7540a58a-294f-455a-a0d2-f9cc7533da06 (Autodesk Fusion 360 design; units mm, degrees)
Autodesk Fusion 360 part; units mm, degrees
note: some values were not read from the file. Set by a fixed rule: which sketch regions a step uses.
sketch "Sketch1" plane through (0, 0, 0) normal (0, 1, 0) x (1, 0, 0)
  circle A0 centre (0, 0) radius 16.9291
  circle A1 centre (0, 0) radius 19.05
  circle A2 centre (0, 0) radius 15.518342
  circle A3 centre (0, 0) radius 15.90815
  arc A4 (19.001185, -1.362896) -> (-17.460766, -7.617357) centre (0, 0) ccw
  circle A5 centre (0, 0) radius 1.984375
  line L0 (0, 0) -> (19.05, 0) construction
  line L1 (0, 0) -> (-1.386487, -15.847615)
  line L2 (0, 0) -> (-2.762421, -15.66647)
  line L3 (0, 0) -> (-4.117332, -15.366093)
  line L4 (0, 0) -> (-5.440908, -14.948771)
  line L5 (0, 0) -> (-6.723075, -14.417681)
  line L6 (0, 0) -> (-7.954075, -13.776862)
  line L7 (0, 0) -> (-9.12454, -13.031194)
  line L8 (-1.386487, -15.847615) -> (-0.003521, -15.968609) construction
  line L9 (-2.762421, -15.66647) -> (-0.028107, -16.148603) construction
  line L10 (-4.117332, -15.366093) -> (-0.094498, -16.444008) construction
  line L11 (-5.440908, -14.948771) -> (-0.222802, -16.848007) construction
  line L12 (-6.723075, -14.417681) -> (-0.432175, -17.351175) construction
  line L13 (-7.954075, -13.776862) -> (-0.740527, -17.941606) construction
  line L14 (-9.12454, -13.031194) -> (-1.164237, -18.605058) construction
  line L15 (0, 0) -> (-10.225562, -12.18635)
  line L16 (-10.225562, -12.18635) -> (-1.717885, -19.325139) construction
  line L17 (0, 0) -> (-11.248761, -11.248761)
  line L18 (-11.248761, -11.248761) -> (-2.414005, -20.083517) construction
  spline S0 degree 5 poles (-2.414005, -20.083517) (-2.349665, -19.980996) (-2.230567, -19.793882) (-2.080667, -19.566991) (-1.93568, -19.366998) (-1.829859, -19.256936) (-1.777433, -19.24436) (-1.753879, -19.282002) (-1.7358, -19.324778) (-1.704144, -19.335998) (-1.648441, -19.295533) (-1.567325, -19.200824) (-1.465447, -19.060921) (-1.351426, -18.892521) (-1.235328, -18.715103) (-1.126503, -18.546748) (-1.03091, -18.398969) (-0.949854, -18.274284) (-0.881626, -18.169398) (-0.822514, -18.077168) (-0.768088, -17.989118) (-0.714277, -17.897515) (-0.658769, -17.798118) (-0.601332, -17.690763) (-0.543004, -17.577752) (-0.485596, -17.462828) (-0.431066, -17.349923) (-0.380956, -17.241995) (-0.33579, -17.139839) (-0.295356, -17.042769) (-0.258972, -16.949298) (-0.225752, -16.857826) (-0.194871, -16.767291) (-0.165849, -16.677925) (-0.138532, -16.590808) (-0.113031, -16.50728) (-0.08968, -16.428431) (-0.068993, -16.354474) (-0.051586, -16.284426) (-0.0379, -16.217121) (-0.027934, -16.152067) (-0.021002, -16.09031) (-0.015408, -16.035467) (-0.009419, -15.991616) (-0.002243, -15.961155) (0.004811, -15.942305) (0.007182, -15.930712) (0.005274, -15.920499) (0.002079, -15.91247) (0, -15.90815) knots 0 0 0 0 0 0 0.02222222 0.04444444 0.06666667 0.08888889 0.11111111 0.13333333 0.15555556 0.17777778 0.2 0.22222222 0.24444444 0.26666667 0.28888889 0.31111111 0.33333333 0.35555556 0.37777778 0.4 0.42222222 0.44444444 0.46666667 0.48888889 0.51111111 0.53333333 0.55555556 0.57777778 0.6 0.62222222 0.64444444 0.66666667 0.68888889 0.71111111 0.73333333 0.75555556 0.77777778 0.8 0.82222222 0.84444444 0.86666667 0.88888889 0.91111111 0.93333333 0.95555556 0.97777778 1 1 1 1 1 1
  line L19 (-2.713358, -20.560516) -> (-2.114652, -19.606519)
  line L20 (0.076308, -16.066729) -> (-0.076308, -15.749572)
  line L21 (-0.251333, -16.927234) -> (0, 0)
  line L22 (0, 0) -> (-0.533009, -6.623728) construction
  line L23 (0, -15.90815) -> (0, 0) construction
  spline S1 degree 5 poles (0, -15.90815) (0, -15.908047) (0, -15.929888) (0, -16.028709) (0, -16.252479) (0, -16.479407) (0, -16.407288) (0, -16.086728) (0, -15.731426) (0, -15.518342) knots 0 0 0 0 0 0 0.2 0.4 0.6 0.8 1 1 1 1 1 1
  spline S2 degree 5 poles (-2.543774, -15.703454) (-2.543757, -15.703352) (-2.54725, -15.724912) (-2.563052, -15.822461) (-2.598834, -16.043352) (-2.63512, -16.26736) (-2.623588, -16.196169) (-2.572329, -15.879734) (-2.515515, -15.529003) (-2.481442, -15.318661) knots 0 0 0 0 0 0 0.2 0.4 0.6 0.8 1 1 1 1 1 1
  line L24 (0, -15.908493) -> (0, -15.907807)
  line L25 (0, -16.224416) -> (0, -14.812267)
  line L26 (-2.543829, -15.703792) -> (-2.543719, -15.703115)
  line L27 (-2.594346, -16.01565) -> (-2.368538, -14.621672)
  spline S3 degree 5 poles (-0.828488, -20.211103) (-0.875607, -20.099613) (-0.963252, -19.895862) (-1.074942, -19.647922) (-1.186084, -19.427318) (-1.272944, -19.301751) (-1.322685, -19.280953) (-1.351955, -19.314345) (-1.376641, -19.35368) (-1.409684, -19.359693) (-1.4582, -19.310841) (-1.523128, -19.204381) (-1.601324, -19.049987) (-1.68695, -18.865522) (-1.773184, -18.671822) (-1.853688, -18.488232) (-1.92442, -18.327069) (-1.984496, -18.191026) (-2.035074, -18.07658) (-2.078678, -17.976085) (-2.118324, -17.880465) (-2.156795, -17.781437) (-2.195695, -17.674442) (-2.235226, -17.559284) (-2.274733, -17.4384) (-2.313026, -17.315776) (-2.348799, -17.195603) (-2.381007, -17.081052) (-2.409257, -16.972988) (-2.433648, -16.870701) (-2.454618, -16.772615) (-2.472784, -16.677008) (-2.488791, -16.5827) (-2.503149, -16.489843) (-2.516184, -16.39948) (-2.528, -16.312949) (-2.538443, -16.23138) (-2.547038, -16.155066) (-2.55302, -16.083137) (-2.555767, -16.014509) (-2.555203, -15.948698) (-2.55217, -15.886628) (-2.548923, -15.831596) (-2.547823, -15.787351) (-2.550035, -15.756135) (-2.553984, -15.736399) (-2.554471, -15.724577) (-2.550955, -15.7148) (-2.546516, -15.707385) (-2.543774, -15.703454) knots 0 0 0 0 0 0 0.02222222 0.04444444 0.06666667 0.08888889 0.11111111 0.13333333 0.15555556 0.17777778 0.2 0.22222222 0.24444444 0.26666667 0.28888889 0.31111111 0.33333333 0.35555556 0.37777778 0.4 0.42222222 0.44444444 0.46666667 0.48888889 0.51111111 0.53333333 0.55555556 0.57777778 0.6 0.62222222 0.64444444 0.66666667 0.68888889 0.71111111 0.73333333 0.75555556 0.77777778 0.8 0.82222222 0.84444444 0.86666667 0.88888889 0.91111111 0.93333333 0.95555556 0.97777778 1 1 1 1 1 1
  line L28 (-0.609261, -20.729832) -> (-1.047716, -19.692375)
  line L29 (-2.644457, -15.84779) -> (-2.443091, -15.559117)
  point P0 (-0.251333, -16.927234)
  point P1 (0, -15.518342)
  point P2 (-1.394384, -19.351171)
  point P3 (-1.825764, -18.551825)
  point P4 (-2.137933, -17.829158)
  point P5 (-2.347905, -17.197017)
  point P6 (-2.474125, -16.666843)
  point P7 (-2.536177, -16.247527)
  point P8 (-2.554479, -15.945307)
  point P9 (-2.549966, -15.763697)
  point P10 (-2.481442, -15.318661)
  dimension "d2" = 55.118
  dimension "id" = 46.566667
  dimension "BaseDiameter" = 47.736385
  dimension "d1" = 3.96875
  dimension "d34" = 5
  dimension "d35" = 5
  dimension "d36" = 5
  dimension "d37" = 5
  dimension "d38" = 5
  dimension "d39" = 5
  dimension "d41" = 2.082893
  dimension "d42" = 4.165785
  dimension "d43" = 6.248678
  dimension "d44" = 8.331571
  dimension "d45" = 10.414464
  dimension "d46" = 12.497356
  dimension "d47" = 14.580249
  dimension "d48" = 5
  dimension "d49" = 16.663142
  dimension "d50" = 5
  dimension "d51" = 18.746035
  dimension "d55" = 3.75
  dimension "d60" = 5
  constraint coincident A0.centre A1.centre
  constraint concentric A0 A2
  constraint horizontal L0
  constraint coincident A4 L0.end
  constraint tangent A3 L8
  constraint tangent A3 L9
  constraint tangent A3 L10
  constraint tangent A3 L11
  constraint tangent A3 L12
  constraint tangent A3 L13
  constraint tangent A3 L14
  constraint tangent A3 L16
  constraint tangent A3 L18
  constraint vertical L24
  constraint vertical L25
  measures "d1" diameter of A5
  measures "d34" angle of L1 L2
  measures "d35" angle of L2 L3
  measures "d36" angle of L3 L4
  measures "d37" angle of L4 L5
  measures "d38" angle of L5 L6
  measures "d39" angle of L6 L7
  measures "d48" angle of L7 L15
  measures "d50" angle of L15 L17
  measures "d55" angle of L21 L22
  measures "d60" angle of L1 L23
extrude "Extrude1" add sketch "Sketch1" along normal blind 304.8 contours A0 A1 S0 S3 | A3 S0 L21 S1 L25 | S2 L27 S3 | A0 A3 L21 S2 L27 S3 | S0 S1 L25 | A2 A3 L21 S1 L25 | A2 A3 L1 L21 | A2 A3 L1 S2 L27 picked at (-1.476298, -18.199938) picked at (-0.183968, -16.389387) picked at (-2.547586, -15.721198) picked at (-2.015818, -16.261518) picked at (0.000926, -15.926276) picked at (-0.104327, -15.777826) picked at (-0.362204, -15.77303) picked at (-1.504128, -15.7053) makes body 1
pattern_circular "C-Pattern2" count 12 over 360 about axis through (0, 1.75, 0) along (0, 1, 0) of bodies 1 makes body 2 at (7.27472, 203.2, 13.707567) makes body 3 at (13.153875, 203.2, 8.233741) makes body 4 at (15.508461, 203.2, 0.553691) makes body 5 at (13.575584, 203.2, -7.518142) makes body 6 at (8.233741, 203.2, -13.153875) makes body 7 at (0.553691, 203.2, -15.508461) makes body 8 at (-7.27472, 203.2, -13.707567) makes body 9 at (-13.153875, 203.2, -8.233741) makes body 10 at (-15.508461, 203.2, -0.553691) makes body 11 at (-13.707567, 203.2, 7.27472) makes body 12 at (-8.233741, 203.2, 13.153875)
extrude "Extrude2" add sketch "Sketch1" along normal blind 304.8 contours A2 A5 L17 L21 | A2 A5 L1 L21 | A2 A5 L1 L2 | A2 A5 L2 L3 | A2 A5 L15 L17 | A2 A5 L3 L4 | A2 A5 L4 L5 | A2 A5 L5 L6 | A2 A5 L6 L7 | A2 A5 L7 L15 picked at (-9.85991, 4.826942) picked at (-0.569669, -10.991468) picked at (-1.625119, -10.885605) picked at (-2.059132, -10.811518) picked at (-7.203577, -8.320903) picked at (-2.993582, -10.590912) picked at (-4.202871, -10.171766) picked at (-5.073405, -9.766755) picked at (-5.632708, -9.455239) picked at (-6.707572, -8.725676) bodies 1 2 3 4 5 6 7 8 9 10 11 12
ref_plane "WorkPlane1" through (6.274689, 152.4, -0.826079) normal (0.130526, 0, 0.991445) x (0.991445, 0, -0.130526)
fillet "Fillet1" [suppressed]
mirror "Mirror3" [suppressed]
pattern_circular "C-Pattern1" [suppressed]
equation "d = 2 in"
equation "OutsideDiameter = d2"
equation "PitchDiameter = d"
equation "id = PitchDiameter - 2 * ( PitchDiameter / TeethNumber )"
equation "BaseDiameter = PitchDiameter * cos(20 deg)"
equation "Length = 12 in"
equation "t = 24"
equation "ShaftDiameter = d1"
equation "TeethNumber = t"
equation "Pitch = 32"
equation "d30 = ( 1.25 * ( PitchDiameter / TeethNumber ) ) - ( PitchDiameter / TeethNumber )"
equation "Basecircum = PI * PitchDiameter * cos(20 deg)"
equation "d41 = Basecircum * 5 / 360"
equation "d42 = Basecircum * 10 / 360"
equation "d43 = Basecircum * 15 / 360"
equation "d44 = Basecircum * 20 / 360"
equation "d45 = Basecircum * 25 / 360"
equation "d46 = Basecircum * 30 / 360"
equation "d47 = Basecircum * 35 / 360"
equation "d49 = Basecircum * 40 / 360"
equation "d51 = Basecircum * 45 / 360"
equation "d55 = ( 360 / ( 4 * TeethNumber ) ) * 1 deg"
